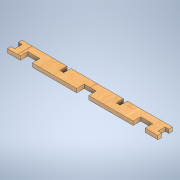
# Autodesk Inventor part: HolzServoHalterHochLang
Saved by Autodesk Inventor 2020.3 (Build 243373010, 373A)
## iProperties
Created: 2020-12-10
Part Number: HolzServoHalterHochLang
Material: Generisch
Document SubType Name: Modeling
Designer: Stefan
Density: 1 g/cm^3
Appearance: Vorgabe
Author: Stefan
Autodesk Inventor part; units mm, degrees
ref_plane "YZ Plane" through (0, 0, 0) normal (1, 0, 0) x (0, 1, 0)
ref_plane "XZ Plane" through (0, 0, 0) normal (0, 1, 0) x (-1, 0, 0)
ref_plane "XY Plane" through (0, 0, 0) normal (0, 0, 1) x (1, 0, 0)
sketch "Skizze1" plane through (0, 0, 0) normal (0, 1, 0) x (-1, 0, 0)
  line L0 (0, 28.875) -> (-10, 28.875)
  line L1 (-10, 28.875) -> (-10, 9.625)
  line L2 (-10, 9.625) -> (0, 9.625)
  line L3 (0, 38.5) -> (0, 28.875)
  line L4 (0, 9.625) -> (0, 0)
  line L5 (-400, 28.875) -> (-390, 28.875)
  line L6 (-390, 28.875) -> (-390, 9.625)
  line L7 (-390, 9.625) -> (-400, 9.625)
  line L8 (-400, 0) -> (-400, 9.625)
  line L9 (-400, 28.875) -> (-400, 38.5)
  line L10 (-120, 19.25) -> (-130, 19.25)
  line L11 (-130, 19.25) -> (-130, 0)
  line L12 (-120, 0) -> (-120, 19.25)
  line L13 (-270, 19.25) -> (-280, 19.25)
  line L14 (-280, 19.25) -> (-280, 0)
  line L15 (-270, 0) -> (-270, 19.25)
  line L16 (-66, 38.5) -> (-66, 18.5)
  line L17 (-66, 18.5) -> (-34, 18.5)
  line L18 (-34, 18.5) -> (-34, 38.5)
  line L19 (-34, 38.5) -> (0, 38.5)
  line L20 (-334, 38.5) -> (-334, 18.5)
  line L21 (-334, 18.5) -> (-366, 18.5)
  line L22 (-366, 18.5) -> (-366, 38.5)
  line L23 (-400, 38.5) -> (-366, 38.5)
  line L24 (-216, 38.5) -> (-216, 18.5)
  line L25 (-216, 18.5) -> (-184, 18.5)
  line L26 (-184, 18.5) -> (-184, 38.5)
  line L27 (-334, 38.5) -> (-216, 38.5)
  line L28 (-184, 38.5) -> (-66, 38.5)
  line L29 (-280, 0) -> (-400, 0)
  line L30 (0, 0) -> (-120, 0)
  line L31 (-130, 0) -> (-270, 0)
  dimension "d0" = 38.5
  dimension "d1" = 400
  dimension "d2" = 10
  dimension "d3" = 19.25
  dimension "d5" = 10
  dimension "d6" = 19.25
  dimension "d8" = 10
  dimension "d9" = 19.25
  dimension "d10" = 10
  dimension "d11" = 19.25
  dimension "d14" = 110
  dimension "d15" = 110
  dimension "d19" = 32
  dimension "d20" = 20
  dimension "d21" = 34
  dimension "d22" = 10
  dimension "d23" = 32
  dimension "d24" = 20
  dimension "d25" = 10
  dimension "d26" = 34
  dimension "d27" = 32
  dimension "d28" = 20
  dimension "d29" = 184
  dimension "d30" = 20
  dimension "d32" = 20
  dimension "d35" = 20
  constraints: 64 end point, 23 parallel, 10 perpendicular, 7 horizontal
  measures "d0" distance of L8.start L9.end
  measures "d1" distance of L9.end L3.start
  measures "d2" distance of L2.end L1.end
  measures "d3" distance of L1.end L0.end
  measures "d5" distance of L6.end L7.end
  measures "d6" distance of L5.end L6.end
  measures "d8" distance of L12.start L11.end
  measures "d9" distance of L11.end L10.end
  measures "d10" distance of L15.start L14.end
  measures "d11" distance of L14.end L13.end
  measures "d14" distance between parallel lines of L6 L14
  measures "d15" distance between parallel lines of L1 L12
  measures "d19" distance of L17.end L16.end
  measures "d20" distance of L16.start L16.end
  measures "d21" distance between parallel lines of L3 L18
  measures "d22" distance between parallel lines of L1 L3
  measures "d23" distance of L20.end L21.end
  measures "d24" distance of L20.start L20.end
  measures "d25" distance of L5.start L5.end
  measures "d26" distance between parallel lines of L9 L22
  measures "d27" distance of L25.end L24.end
  measures "d28" distance of L24.end L24.start
  measures "d29" distance between parallel lines of L3 L26
  measures "d30" distance of L25.end L26.end
  measures "d32" distance of L21.end L22.end
  measures "d35" distance of L17.end L18.end
extrude "Extrusion1" add sketch "Skizze1" along normal blind 10
